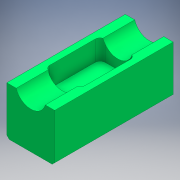
# Autodesk Inventor part: Semi cuscinetto 2
Saved by Autodesk Inventor 2016 (Build 200138000, 138)
## iProperties
Created: 2016-09-10
Part Number: Semi cuscinetto 2
Material: Generic
Document SubType Name: Modeling
Designer: Muhammad
Density: 1 g/cm^3
Appearance: Default
Author: Muhammad
Autodesk Inventor part; units mm, degrees
ref_plane "YZ Plane" through (0, 0, 0) normal (1, 0, 0) x (0, 1, 0)
ref_plane "XZ Plane" through (0, 0, 0) normal (0, 1, 0) x (-1, 0, 0)
ref_plane "XY Plane" through (0, 0, 0) normal (0, 0, 1) x (1, 0, 0)
sketch "Sketch1" plane through (0, 0, 0) normal (0, 1, 0) x (-1, 0, 0)
  line L0 (-9.5, 9.5) -> (9.5, 9.5)
  line L1 (9.5, 9.5) -> (9.5, -9.5)
  line L2 (9.5, -9.5) -> (-9.5, -9.5)
  line L3 (-9.5, -9.5) -> (-9.5, 9.5)
  line L4 (-9.5, 9.5) -> (9.5, -9.5) construction
  line L5 (9.5, 9.5) -> (-9.5, -9.5) construction
  point P0 (0, 0)
  constraints: 12 end point, 2 midpoint, 2 parallel, 1 horizontal, 1 perpendicular
extrude "Extrusion1" add sketch "Sketch1" along normal blind 47
sketch "Sketch2" plane through (-9.5, 0, 9.5) normal (0, 0, 1) x (1, 0, 0)
  line L0 (0, 47) -> (19, 47) construction
  line L1 (9.5, 34.5) -> (9.5, 12.5) construction
  line L2 (2.5, 34.5) -> (16.5, 34.5)
  line L3 (16.5, 34.5) -> (16.5, 12.5)
  line L4 (16.5, 12.5) -> (2.5, 12.5)
  line L5 (2.5, 12.5) -> (2.5, 34.5)
  line L6 (2.5, 34.5) -> (16.5, 12.5) construction
  line L7 (16.5, 34.5) -> (2.5, 12.5) construction
  point P0 (9.5, 0)
  point P1 (9.5, 23.5)
  dimension "d5" = 22
  dimension "d6" = 14
  dimension "d7" = 22
  constraints: 14 end point, 3 midpoint, 2 parallel, 1 horizontal, 1 perpendicular, 1 vertical
  measures "d5" distance of L1.start L1.end
  measures "d6" distance of L3.end L4.end
  measures "d7" distance of L2.end L3.end
extrude "Extrusion2" cut sketch "Sketch2" against normal blind 8
fillet "Fillet1" radius 2 4 edges at (-7, 34.5, 5.5) (-7, 12.5, 5.5) (7, 34.5, 5.5) (7, 12.5, 5.5)
sketch "Sketch3" plane through (0, 47, 0) normal (0, 1, 0) x (1, 0, 0)
  line L0 (9.5, 9.5) -> (-9.5, 9.5) construction
  line L1 (0, 9.5) -> (0, -11.2) construction
  circle A0 centre (0, -11.2) radius 6
  point P0 (0, 0)
  dimension "d11" = 20.7
  dimension "d12" = 12
  constraints: 2 end point, 1 centre point, 1 coincident, 1 midpoint, 1 vertical
  measures "d11" distance of L1.start L1.end
  measures "d12" diameter of A0
extrude "Extrusion3" cut sketch "Sketch3" against normal through all
chamfer "Chamfer1" distance 1 angle 45 2 edges at (-9.5, 23.5, -9.5) (9.5, 23.5, -9.5)
body "Solid1"
